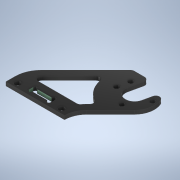
# Autodesk Inventor part: Shoulder_side_frame
Saved by Autodesk Inventor 2022.3 (Build 263350000, 350)
## iProperties
Part Number: Shoulder_side_frame
Material: アルミニウム 2014-T4
Document SubType Name: Modeling
Designer: Masato Kubotera
Density: 2.8 g/cm^3
Appearance: 光沢 - 黒
Description: A2017 T2
Mass: 4.81119 g
Surface Area: 23.7102 cm^2
Volume: 1.71828 cm^3
Author: Masato Kubotera
Autodesk Inventor part; units mm, degrees
ref_plane "YZ Plane" through (0, 0, 0) normal (1, 0, 0) x (0, 1, 0)
ref_plane "XZ Plane" through (0, 0, 0) normal (0, 1, 0) x (-1, 0, 0)
ref_plane "XY Plane" through (0, 0, 0) normal (0, 0, 1) x (1, 0, 0)
sketch "スケッチ1" plane through (0, 0, 0) normal (1, 0, 0) x (0, 1, 0)
  line L0 (-29.3, 41) -> (-29.3, 9)
  line L1 (-29.3, 25) -> (-24.3, 25) construction
  line L2 (-26.8, 31) -> (-24.3, 31) construction
  line L3 (-24.3, 31) -> (-24.3, 19) construction
  line L4 (-24.3, 19) -> (-26.8, 19) construction
  line L5 (-26.8, 19) -> (-26.8, 31) construction
  line L6 (-26.8, 31) -> (-24.3, 19) construction
  line L7 (-24.3, 31) -> (-26.8, 19) construction
  circle A0 centre (-26.8, 37) radius 1.6
  line L8 (-26.8, 70.0011) -> (-26.8, -20.0011) construction
  line L9 (-29.3, 41) -> (-24.3, 41)
  circle A1 centre (0, 0) radius 5.05
  line L10 (-1.476, 8.3709) -> (1.476, -8.3709) construction
  circle A2 centre (-1.476, 8.3709) radius 1.35
  arc A3 (-7.6162, -7.6162) -> (10.7709, 0) centre (0, 0) ccw
  line L11 (-26.85, 31.05) -> (-24.25, 31.05)
  line L12 (-24.25, 31.05) -> (-24.25, 18.95)
  line L13 (-24.25, 18.95) -> (-26.85, 18.95)
  line L14 (-26.85, 18.95) -> (-26.85, 31.05)
  line L15 (-26.85, 31.05) -> (-24.25, 18.95) construction
  line L16 (-24.25, 31.05) -> (-26.85, 18.95) construction
  arc A4 (-24.25, 28.95) -> (-24.25, 31.05) centre (-24.25, 30) ccw
  line L17 (-25.55, 31) -> (-25.55, 19) construction
  arc A5 (-26.85, 31.05) -> (-26.85, 28.95) centre (-26.85, 30) ccw
  arc A6 (-24.25, 18.95) -> (-24.25, 21.05) centre (-24.25, 20) ccw
  arc A7 (-26.85, 21.05) -> (-26.85, 18.95) centre (-26.85, 20) ccw
  circle A8 centre (-26.8, 13) radius 1.6
  line L18 (-14.1813, 36.8087) -> (10.7709, 11.8566)
  line L19 (10.7709, 11.8566) -> (10.7709, 0)
  line L20 (-20.6489, 5.4166) -> (-7.6162, -7.6162)
  circle A9 centre (-6.9628, 4.8754) radius 1.35
  circle A10 centre (-8.3709, -1.476) radius 1.35
  circle A11 centre (0, 0) radius 16 construction
  arc A12 (-14.1813, 36.8087) -> (-24.3, 41) centre (-24.3, 26.6899) ccw
  line L21 (-20.3, 36.1924) -> (-20.3, 10.2769)
  arc A13 (-17.0097, 33.9803) -> (-20.3, 36.1924) centre (-24.3, 26.6899) ccw
  line L22 (6.7709, 10.0706) -> (6.7709, 8.438)
  circle A14 centre (-1.476, 8.3709) radius 2.4 construction
  line L23 (1.002, 15.9686) -> (-17.0097, 33.9803)
  arc A15 (-20.6489, 5.4166) -> (-29.3, 9) centre (-29.3, -3.2345) ccw
  circle A16 centre (-4.8754, -6.9628) radius 1.35
  circle A17 centre (1.476, -8.3709) radius 1.35
  arc A18 (-17.8205, 8.245) -> (-20.3, 10.2769) centre (-29.3, -3.2345) ccw
  line L24 (-1.093, -4.9303) -> (8.1951, -6.9894)
  line L25 (1.093, 4.9303) -> (10.7709, 2.7848)
  circle A19 centre (6.9628, -4.8754) radius 1.35
  circle A20 centre (8.3709, 1.476) radius 1.35
  circle A21 centre (4.8754, 6.9628) radius 1.35
  circle A22 centre (-6.9628, 4.8754) radius 2.4 construction
  circle A23 centre (-8.3709, -1.476) radius 2.4 construction
  circle A24 centre (-4.8754, -6.9628) radius 2.4 construction
  circle A25 centre (1.476, -8.3709) radius 2.4 construction
  circle A26 centre (6.9628, -4.8754) radius 2.4 construction
  circle A27 centre (8.3709, 1.476) radius 2.4 construction
  circle A28 centre (4.8754, 6.9628) radius 2.4 construction
  line L26 (6.9628, -4.8754) -> (8.3709, 1.476) construction
  line L27 (-17.8205, 8.245) -> (-15.0385, 5.463)
  arc A29 (1.002, 15.9686) -> (-15.0385, 5.463) centre (0, 0) ccw
  point P0 (-25.55, 25)
  point P1 (-26.8, 25)
  point P2 (-24.25, 21.05)
  point P3 (-26.85, 21.05)
  point P4 (-26.85, 28.95)
  point P5 (-0.8769, 4.9733)
  point P6 (0.8769, -4.9733)
  dimension "d0" = 5
  dimension "d1" = 32
  dimension "d2" = 2.5
  dimension "d3" = 12
  dimension "d4" = 3.2
  dimension "d5" = 5
  dimension "d6" = 10.1
  dimension "d7" = 17
  dimension "d8" = 2.7
  dimension "d10" = 29.3
  dimension "d11" = 1.05
  dimension "d12" = 0.05
  dimension "d13" = 0.05
  dimension "d14" = 24
  dimension "d15" = 25
  dimension "d19" = 360
  dimension "d23" = 32
  dimension "d24" = 45
  dimension "d31" = 4
  dimension "d32" = 4
  dimension "d37" = 4.8
  dimension "d46" = 4
  dimension "d47" = 4
  dimension "d53" = 360
  dimension "d56" = 10
  constraints: 54 end point, 30 centre point, 29 point on circle, 11 midpoint, 10 tangent, 8 coincident, 8 parallel, 7 point on line, 7 symmetric about line, 3 horizontal, 3 perpendicular, 3 vertical, 1 concentric, 1 line through centre, 42 other
  measures "d0" distance of L1.end L1.start
  measures "d1" distance of L0.start L0.end
  measures "d2" distance of L3.end L4.end
  measures "d3" distance of L2.end L3.end
  measures "d4" diameter of A0
  measures "d5" distance of L0.start A12.end
  measures "d6" diameter of A1
  measures "d7" distance of L10.start L10.end
  measures "d8" diameter of A2
  measures "d10" horizontal distance of A1.centre L0.end
  measures "d11" radius of A4
  measures "d12" distance between parallel lines of L2 L11
  measures "d13" distance between parallel lines of L3 L12
  measures "d14" distance of A8.centre A0.centre
  measures "d15" vertical distance of A1.centre L1.start
  measures "d23" diameter of A11
  measures "d24" angle of L0 L18
  measures "d31" distance between parallel lines of L19 L22
  measures "d32" distance between parallel lines of L21 L3
  measures "d37" diameter of A14
  measures "d46" distance between parallel lines of L23 L18
  measures "d47" distance of L20.start L27.start
  measures "d56" angle of L10 L19
extrude "押し出し1" add sketch "スケッチ1" along normal blind 2 contours L9 A12 L18 L19 L25 A1 L24 A3 L20 A15 L0 | A9 | A16
fillet "フィレット1" radius 2 4 edges at (1, -20.3, 36.1924) (1, -20.3, 10.2769) (1, -15.0385, 5.463) (1, 1.002, 15.9686)
fillet "フィレット2" radius 2 3 edges at (1, 10.7709, 11.8566) (1, 8.1951, -6.9894) (1, 10.7709, 2.7848)
equation "\"d13\" = d12"
